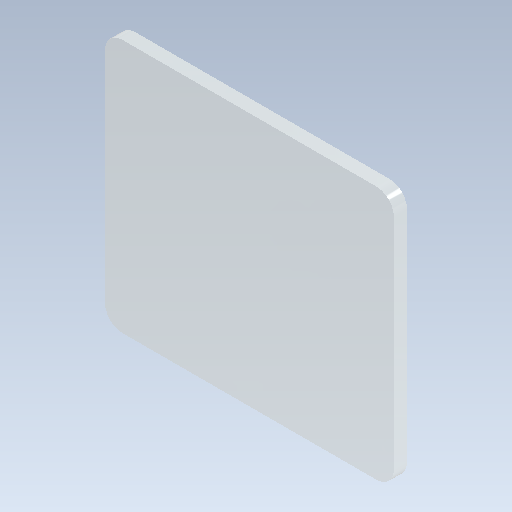
# Autodesk Inventor part: Ventana
Saved by Autodesk Inventor 2020.1 (Build 241239000, 239)
## iProperties
Created: 2019-12-09
Part Number: Ventana
Material: Glass
Document SubType Name: Modeling
Designer: Daniel
Density: 2.18 g/cm^3
Appearance: Clear
Author: Daniel
Autodesk Inventor part; units mm, degrees
ref_plane "YZ Plane" through (0, 0, 0) normal (1, 0, 0) x (0, 1, 0)
ref_plane "XZ Plane" through (0, 0, 0) normal (0, 1, 0) x (-1, 0, 0)
ref_plane "XY Plane" through (0, 0, 0) normal (0, 0, 1) x (1, 0, 0)
sketch "Sketch1" plane through (0, 0, 0) normal (0, 0, 1) x (1, 0, 0)
  line L0 (29, -1.9786) -> (-29, -1.9786) projected
  arc A0 (29, -1.9786) -> (33, 2.0214) centre (29, 2.0214) ccw projected
  line L1 (33, 52.0214) -> (33, 2.0214) projected
  arc A1 (33, 52.0214) -> (29, 56.0214) centre (29, 52.0214) ccw projected
  line L2 (-29, 56.0214) -> (29, 56.0214) projected
  arc A2 (-29, 56.0214) -> (-33, 52.0214) centre (-29, 52.0214) ccw projected
  line L3 (-33, 2.0214) -> (-33, 52.0214) projected
  arc A3 (-33, 2.0214) -> (-29, -1.9786) centre (-29, 2.0214) ccw projected
  point P0 (0, 0)
ref_plane "Work Plane1" through (-87, -150, -3) normal (0, 0, -1) x (0, 1, 0)
extrude "Extrusion1" add sketch "Sketch1" against normal up to surface (3 mm away)
body "Solid1"
